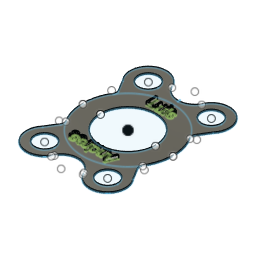
2D Plancha #1 (Autodesk Fusion 360 design; units mm, degrees)
Autodesk Fusion 360 part; units mm, degrees
sketch "Boceto1" plane through (0, 0, 0) normal (0, 0, 1) x (1, 0, 0)
  circle A0 centre (-31.4946, 51.8022) radius 10
  arc A1 (-14.8964, 58.7663) -> (-45.1155, 40.0347) centre (-31.4946, 51.8022) ccw
  line L0 (-45.1155, 40.0347) -> (-38.2984, 28.8221)
  arc A2 (-38.3137, 23.6021) -> (-38.2984, 28.8221) centre (-42.5708, 26.2246) ccw
  arc A3 (38.2984, 28.8221) -> (38.3137, 23.6021) centre (42.5708, 26.2246) ccw
  line L1 (45.1155, 40.0347) -> (38.2984, 28.8221)
  arc A4 (45.1155, 40.0347) -> (14.8964, 58.7663) centre (31.4946, 51.8022) ccw
  circle A5 centre (31.4946, 51.8022) radius 10
  arc A6 (-15.8954, 60.7834) -> (15.8954, 60.7834) centre (0, 66.8115) ccw
  line L2 (0, 49.8115) -> (0, 51.8022)
  line L3 (0, 49.8115) -> (0, 51.8022)
  arc A7 (45, 0) -> (-45, 0) centre (0, 0) ccw
  arc A8 (27.5, 0) -> (-27.5, 0) centre (0, 0) ccw
  arc A9 (-45, 0) -> (45, 0) centre (0, 0) ccw
  arc A10 (-27.5, 0) -> (27.5, 0) centre (0, 0) ccw
  line L4 (-45.1155, -40.0347) -> (-38.2984, -28.8221)
  arc A11 (-38.2984, -28.8221) -> (-38.3137, -23.6021) centre (-42.5708, -26.2246) ccw
  arc A12 (-45.1155, -40.0347) -> (-14.8964, -58.7663) centre (-31.4946, -51.8022) ccw
  circle A13 centre (-31.4946, -51.8022) radius 10
  arc A14 (15.8954, -60.7834) -> (-15.8954, -60.7834) centre (0, -66.8115) ccw
  arc A15 (14.8964, -58.7663) -> (45.1155, -40.0347) centre (31.4946, -51.8022) ccw
  circle A16 centre (31.4946, -51.8022) radius 10
  line L5 (45.1155, -40.0347) -> (38.2984, -28.8221)
  arc A17 (38.3137, -23.6021) -> (38.2984, -28.8221) centre (42.5708, -26.2246) ccw
  line L6 (-12.0362, 30.2431) -> (-12.0909, 40.2429)
  line L7 (-12.0909, 40.2429) -> (-10.7676, 40.2502)
  line L8 (-10.7676, 40.2502) -> (-10.7193, 31.4304)
  line L9 (-10.7193, 31.4304) -> (-5.7944, 31.4573)
  line L10 (-5.7944, 31.4573) -> (-5.788, 30.2773)
  line L11 (-5.788, 30.2773) -> (-12.0362, 30.2431)
  line L12 (0.3784, 30.311) -> (0.3726, 31.3751)
  spline S0 degree 2 poles (0.3726, 31.3751) (-0.4665, 30.1427) (-1.9195, 30.1347) knots 0 0 0 1 1 1
  spline S1 degree 2 poles (-1.9195, 30.1347) (-2.5606, 30.1312) (-3.1179, 30.3737) knots 0 0 0 1 1 1
  spline S2 degree 2 poles (-3.1179, 30.3737) (-3.6752, 30.6162) (-3.9467, 30.9865) knots 0 0 0 1 1 1
  spline S3 degree 2 poles (-3.9467, 30.9865) (-4.2181, 31.3568) (-4.3302, 31.8951) knots 0 0 0 1 1 1
  spline S4 degree 2 poles (-4.3302, 31.8951) (-4.4072, 32.2562) (-4.4115, 33.0406) knots 0 0 0 1 1 1
  line L13 (-4.4115, 33.0406) -> (-4.4361, 37.529)
  line L14 (-4.4361, 37.529) -> (-3.2083, 37.5357)
  line L15 (-3.2083, 37.5357) -> (-3.1863, 33.518)
  spline S5 degree 2 poles (-3.1863, 33.518) (-3.181, 32.5562) (-3.1042, 32.2224) knots 0 0 0 1 1 1
  spline S6 degree 2 poles (-3.1042, 32.2224) (-2.9855, 31.7387) (-2.6089, 31.4645) knots 0 0 0 1 1 1
  spline S7 degree 2 poles (-2.6089, 31.4645) (-2.2322, 31.1903) (-1.6797, 31.1933) knots 0 0 0 1 1 1
  spline S8 degree 2 poles (-1.6797, 31.1933) (-1.1272, 31.1964) (-0.6444, 31.4821) knots 0 0 0 1 1 1
  spline S9 degree 2 poles (-0.6444, 31.4821) (-0.1617, 31.7678) (0.0369, 32.2566) knots 0 0 0 1 1 1
  spline S10 degree 2 poles (0.0369, 32.2566) (0.2355, 32.7454) (0.2304, 33.6731) knots 0 0 0 1 1 1
  line L16 (0.2304, 33.6731) -> (0.2092, 37.5544)
  line L17 (0.2092, 37.5544) -> (1.437, 37.5611)
  line L18 (1.437, 37.5611) -> (1.4766, 30.317)
  line L19 (1.4766, 30.317) -> (0.3784, 30.311)
  line L20 (3.36, 38.9154) -> (3.3523, 40.3274)
  line L21 (3.3523, 40.3274) -> (4.5801, 40.3341)
  line L22 (4.5801, 40.3341) -> (4.5878, 38.9221)
  line L23 (4.5878, 38.9221) -> (3.36, 38.9154)
  line L24 (3.407, 30.3276) -> (3.3674, 37.5717)
  line L25 (3.3674, 37.5717) -> (4.5952, 37.5784)
  line L26 (4.5952, 37.5784) -> (4.6348, 30.3343)
  line L27 (4.6348, 30.3343) -> (3.407, 30.3276)
  line L28 (6.0009, 32.5041) -> (7.214, 32.7018)
  spline S11 degree 2 poles (7.214, 32.7018) (7.3203, 31.9725) (7.7897, 31.5862) knots 0 0 0 1 1 1
  spline S12 degree 2 poles (7.7897, 31.5862) (8.259, 31.2) (9.098, 31.2045) knots 0 0 0 1 1 1
  spline S13 degree 2 poles (9.098, 31.2045) (9.9439, 31.2092) (10.3513, 31.5559) knots 0 0 0 1 1 1
  spline S14 degree 2 poles (10.3513, 31.5559) (10.7586, 31.9026) (10.7561, 32.3664) knots 0 0 0 1 1 1
  spline S15 degree 2 poles (10.7561, 32.3664) (10.7538, 32.7825) (10.391, 33.0193) knots 0 0 0 1 1 1
  spline S16 degree 2 poles (10.391, 33.0193) (10.1377, 33.1816) (9.1336, 33.4285) knots 0 0 0 1 1 1
  spline S17 degree 2 poles (9.1336, 33.4285) (7.7812, 33.7622) (7.258, 34.0083) knots 0 0 0 1 1 1
  spline S18 degree 2 poles (7.258, 34.0083) (6.7348, 34.2544) (6.463, 34.6929) knots 0 0 0 1 1 1
  spline S19 degree 2 poles (6.463, 34.6929) (6.1911, 35.1314) (6.1882, 35.6635) knots 0 0 0 1 1 1
  spline S20 degree 2 poles (6.1882, 35.6635) (6.1856, 36.1478) (6.405, 36.5617) knots 0 0 0 1 1 1
  spline S21 degree 2 poles (6.405, 36.5617) (6.6244, 36.9756) (7.0049, 37.2505) knots 0 0 0 1 1 1
  spline S22 degree 2 poles (7.0049, 37.2505) (7.2902, 37.4635) (7.784, 37.6129) knots 0 0 0 1 1 1
  spline S23 degree 2 poles (7.784, 37.6129) (8.2777, 37.7622) (8.8439, 37.7653) knots 0 0 0 1 1 1
  spline S24 degree 2 poles (8.8439, 37.7653) (9.6965, 37.77) (10.3425, 37.528) knots 0 0 0 1 1 1
  spline S25 degree 2 poles (10.3425, 37.528) (10.9884, 37.2859) (11.2977, 36.8681) knots 0 0 0 1 1 1
  spline S26 degree 2 poles (11.2977, 36.8681) (11.6069, 36.4503) (11.7267, 35.7483) knots 0 0 0 1 1 1
  line L29 (11.7267, 35.7483) -> (10.5271, 35.5781)
  spline S27 degree 2 poles (10.5271, 35.5781) (10.4422, 36.1369) (10.0482, 36.4486) knots 0 0 0 1 1 1
  spline S28 degree 2 poles (10.0482, 36.4486) (9.6543, 36.7602) (8.9381, 36.7563) knots 0 0 0 1 1 1
  spline S29 degree 2 poles (8.9381, 36.7563) (8.0922, 36.7517) (7.7322, 36.47) knots 0 0 0 1 1 1
  spline S30 degree 2 poles (7.7322, 36.47) (7.3723, 36.1884) (7.3743, 35.8132) knots 0 0 0 1 1 1
  spline S31 degree 2 poles (7.3743, 35.8132) (7.3756, 35.5745) (7.5267, 35.3843) knots 0 0 0 1 1 1
  spline S32 degree 2 poles (7.5267, 35.3843) (7.6779, 35.1873) (7.9992, 35.0594) knots 0 0 0 1 1 1
  spline S33 degree 2 poles (7.9992, 35.0594) (8.1837, 34.9922) (9.0855, 34.7516) knots 0 0 0 1 1 1
  spline S34 degree 2 poles (9.0855, 34.7516) (10.3902, 34.4108) (10.9064, 34.192) knots 0 0 0 1 1 1
  spline S35 degree 2 poles (10.9064, 34.192) (11.4226, 33.9731) (11.7183, 33.5518) knots 0 0 0 1 1 1
  spline S36 degree 2 poles (11.7183, 33.5518) (12.0139, 33.1305) (12.0173, 32.5029) knots 0 0 0 1 1 1
  spline S37 degree 2 poles (12.0173, 32.5029) (12.0207, 31.889) (11.6655, 31.3448) knots 0 0 0 1 1 1
  spline S38 degree 2 poles (11.6655, 31.3448) (11.3104, 30.8005) (10.6367, 30.5001) knots 0 0 0 1 1 1
  spline S39 degree 2 poles (10.6367, 30.5001) (9.963, 30.1997) (9.1104, 30.1951) knots 0 0 0 1 1 1
  spline S40 degree 2 poles (9.1104, 30.1951) (7.6984, 30.1873) (6.9551, 30.7699) knots 0 0 0 1 1 1
  spline S41 degree 2 poles (6.9551, 30.7699) (6.2118, 31.3525) (6.0009, 32.5041) knots 0 0 0 1 1 1
  line L30 (20.5732, -29.8279) -> (16.7328, -39.8279)
  line L31 (16.7328, -39.8279) -> (15.3071, -39.8279)
  line L32 (15.3071, -39.8279) -> (11.2144, -29.8279)
  line L33 (11.2144, -29.8279) -> (12.7219, -29.8279)
  line L34 (12.7219, -29.8279) -> (13.8883, -32.8566)
  line L35 (13.8883, -32.8566) -> (18.0697, -32.8566)
  line L36 (18.0697, -32.8566) -> (19.168, -29.8279)
  line L37 (19.168, -29.8279) -> (20.5732, -29.8279)
  line L38 (17.6878, -33.9343) -> (14.2976, -33.9343)
  line L39 (14.2976, -33.9343) -> (15.3412, -36.7038)
  spline S42 degree 2 poles (15.3412, -36.7038) (15.8187, -37.9657) (16.0506, -38.7774) knots 0 0 0 1 1 1
  spline S43 degree 2 poles (16.0506, -38.7774) (16.2416, -37.8156) (16.5895, -36.8675) knots 0 0 0 1 1 1
  line L40 (16.5895, -36.8675) -> (17.6878, -33.9343)
  line L41 (10.3139, -29.8279) -> (10.3139, -37.0721)
  line L42 (10.3139, -37.0721) -> (9.2089, -37.0721)
  line L43 (9.2089, -37.0721) -> (9.2089, -36.0421)
  spline S44 degree 2 poles (9.2089, -36.0421) (8.4108, -37.2358) (6.9033, -37.2358) knots 0 0 0 1 1 1
  spline S45 degree 2 poles (6.9033, -37.2358) (6.2485, -37.2358) (5.6994, -37.0005) knots 0 0 0 1 1 1
  spline S46 degree 2 poles (5.6994, -37.0005) (5.1502, -36.7651) (4.8774, -36.3832) knots 0 0 0 1 1 1
  spline S47 degree 2 poles (4.8774, -36.3832) (4.6045, -36.0012) (4.4954, -35.4759) knots 0 0 0 1 1 1
  spline S48 degree 2 poles (4.4954, -35.4759) (4.4272, -35.1349) (4.4272, -34.2822) knots 0 0 0 1 1 1
  line L44 (4.4272, -34.2822) -> (4.4272, -29.8279)
  line L45 (4.4272, -29.8279) -> (5.655, -29.8279)
  line L46 (5.655, -29.8279) -> (5.655, -34.2345)
  spline S49 degree 2 poles (5.655, -34.2345) (5.655, -34.9848) (5.7983, -35.3566) knots 0 0 0 1 1 1
  spline S50 degree 2 poles (5.7983, -35.3566) (5.9415, -35.7283) (6.3064, -35.95) knots 0 0 0 1 1 1
  spline S51 degree 2 poles (6.3064, -35.95) (6.6714, -36.1717) (7.1625, -36.1717) knots 0 0 0 1 1 1
  spline S52 degree 2 poles (7.1625, -36.1717) (7.947, -36.1717) (8.5165, -35.6737) knots 0 0 0 1 1 1
  spline S53 degree 2 poles (8.5165, -35.6737) (9.0861, -35.1758) (9.0861, -33.7842) knots 0 0 0 1 1 1
  line L47 (9.0861, -33.7842) -> (9.0861, -29.8279)
  line L48 (9.0861, -29.8279) -> (10.3139, -29.8279)
  line L49 (-2.1554, -29.8279) -> (-2.1554, -30.742)
  spline S54 degree 2 poles (-2.1554, -30.742) (-1.4664, -29.6642) (-0.1294, -29.6642) knots 0 0 0 1 1 1
  spline S55 degree 2 poles (-0.1294, -29.6642) (0.7369, -29.6642) (1.4633, -30.1417) knots 0 0 0 1 1 1
  spline S56 degree 2 poles (1.4633, -30.1417) (2.1898, -30.6192) (2.5888, -31.4752) knots 0 0 0 1 1 1
  spline S57 degree 2 poles (2.5888, -31.4752) (2.9879, -32.3313) (2.9879, -33.4432) knots 0 0 0 1 1 1
  spline S58 degree 2 poles (2.9879, -33.4432) (2.9879, -34.5278) (2.6264, -35.4111) knots 0 0 0 1 1 1
  spline S59 degree 2 poles (2.6264, -35.4111) (2.2648, -36.2945) (1.5418, -36.7651) knots 0 0 0 1 1 1
  spline S60 degree 2 poles (1.5418, -36.7651) (0.8187, -37.2358) (-0.0749, -37.2358) knots 0 0 0 1 1 1
  spline S61 degree 2 poles (-0.0749, -37.2358) (-0.7297, -37.2358) (-1.2413, -36.9596) knots 0 0 0 1 1 1
  spline S62 degree 2 poles (-1.2413, -36.9596) (-1.7529, -36.6833) (-2.0735, -36.2399) knots 0 0 0 1 1 1
  line L50 (-2.0735, -36.2399) -> (-2.0735, -39.8279)
  line L51 (-2.0735, -39.8279) -> (-3.2945, -39.8279)
  line L52 (-3.2945, -39.8279) -> (-3.2945, -29.8279)
  line L53 (-3.2945, -29.8279) -> (-2.1554, -29.8279)
  spline S63 degree 2 poles (1.726, -33.4432) (1.726, -32.0516) (1.1393, -31.3627) knots 0 0 0 1 1 1
  spline S64 degree 2 poles (1.1393, -31.3627) (0.5527, -30.6737) (-0.2454, -30.6737) knots 0 0 0 1 1 1
  spline S65 degree 2 poles (-0.2454, -30.6737) (-1.0503, -30.6737) (-1.6131, -31.332) knots 0 0 0 1 1 1
  spline S66 degree 2 poles (-1.6131, -31.332) (-2.1758, -31.9902) (-2.1758, -33.3409) knots 0 0 0 1 1 1
  spline S67 degree 2 poles (-2.1758, -33.3409) (-2.1758, -34.8279) (-1.6028, -35.5237) knots 0 0 0 1 1 1
  spline S68 degree 2 poles (-1.6028, -35.5237) (-1.0298, -36.2194) (-0.1908, -36.2194) knots 0 0 0 1 1 1
  spline S69 degree 2 poles (-0.1908, -36.2194) (0.6277, -36.2194) (1.1768, -35.551) knots 0 0 0 1 1 1
  spline S70 degree 2 poles (1.1768, -35.551) (1.726, -34.8825) (1.726, -33.4432) knots 0 0 0 1 1 1
  line L54 (-5.2113, -29.8279) -> (-5.2113, -37.0721)
  line L55 (-5.2113, -37.0721) -> (-6.3163, -37.0721)
  line L56 (-6.3163, -37.0721) -> (-6.3163, -35.9739)
  spline S71 degree 2 poles (-6.3163, -35.9739) (-6.7393, -36.7447) (-7.0974, -36.9902) knots 0 0 0 1 1 1
  spline S72 degree 2 poles (-7.0974, -36.9902) (-7.4555, -37.2358) (-7.8852, -37.2358) knots 0 0 0 1 1 1
  spline S73 degree 2 poles (-7.8852, -37.2358) (-8.506, -37.2358) (-9.1472, -36.8402) knots 0 0 0 1 1 1
  line L57 (-9.1472, -36.8402) -> (-8.7243, -35.701)
  spline S74 degree 2 poles (-8.7243, -35.701) (-8.274, -35.9671) (-7.8238, -35.9671) knots 0 0 0 1 1 1
  spline S75 degree 2 poles (-7.8238, -35.9671) (-7.4214, -35.9671) (-7.1008, -35.7249) knots 0 0 0 1 1 1
  spline S76 degree 2 poles (-7.1008, -35.7249) (-6.7802, -35.4827) (-6.6438, -35.053) knots 0 0 0 1 1 1
  spline S77 degree 2 poles (-6.6438, -35.053) (-6.4391, -34.3982) (-6.4391, -33.6205) knots 0 0 0 1 1 1
  line L58 (-6.4391, -33.6205) -> (-6.4391, -29.8279)
  line L59 (-6.4391, -29.8279) -> (-5.2113, -29.8279)
  line L60 (-14.8361, -32.1608) -> (-16.1049, -32.0039)
  spline S78 degree 2 poles (-16.1049, -32.0039) (-15.8047, -30.892) (-14.993, -30.2781) knots 0 0 0 1 1 1
  spline S79 degree 2 poles (-14.993, -30.2781) (-14.1813, -29.6642) (-12.9193, -29.6642) knots 0 0 0 1 1 1
  spline S80 degree 2 poles (-12.9193, -29.6642) (-11.33, -29.6642) (-10.3989, -30.643) knots 0 0 0 1 1 1
  spline S81 degree 2 poles (-10.3989, -30.643) (-9.4678, -31.6219) (-9.4678, -33.3886) knots 0 0 0 1 1 1
  spline S82 degree 2 poles (-9.4678, -33.3886) (-9.4678, -35.2167) (-10.4091, -36.2263) knots 0 0 0 1 1 1
  spline S83 degree 2 poles (-10.4091, -36.2263) (-11.3504, -37.2358) (-12.8511, -37.2358) knots 0 0 0 1 1 1
  spline S84 degree 2 poles (-12.8511, -37.2358) (-14.3041, -37.2358) (-15.2249, -36.2467) knots 0 0 0 1 1 1
  spline S85 degree 2 poles (-15.2249, -36.2467) (-16.1458, -35.2576) (-16.1458, -33.4636) knots 0 0 0 1 1 1
  spline S86 degree 2 poles (-16.1458, -33.4636) (-16.1458, -33.3545) (-16.139, -33.1362) knots 0 0 0 1 1 1
  line L61 (-16.139, -33.1362) -> (-10.7365, -33.1362)
  spline S87 degree 2 poles (-10.7365, -33.1362) (-10.8047, -31.9425) (-11.4118, -31.3081) knots 0 0 0 1 1 1
  spline S88 degree 2 poles (-11.4118, -31.3081) (-12.0189, -30.6737) (-12.9262, -30.6737) knots 0 0 0 1 1 1
  spline S89 degree 2 poles (-12.9262, -30.6737) (-13.6015, -30.6737) (-14.079, -31.0284) knots 0 0 0 1 1 1
  spline S90 degree 2 poles (-14.079, -31.0284) (-14.5564, -31.3832) (-14.8361, -32.1608) knots 0 0 0 1 1 1
  line L62 (-10.8047, -34.1458) -> (-14.8498, -34.1458)
  spline S91 degree 2 poles (-14.8498, -34.1458) (-14.7679, -35.0598) (-14.3859, -35.5169) knots 0 0 0 1 1 1
  spline S92 degree 2 poles (-14.3859, -35.5169) (-13.7993, -36.2263) (-12.8648, -36.2263) knots 0 0 0 1 1 1
  spline S93 degree 2 poles (-12.8648, -36.2263) (-12.0189, -36.2263) (-11.4425, -35.6601) knots 0 0 0 1 1 1
  spline S94 degree 2 poles (-11.4425, -35.6601) (-10.8661, -35.0939) (-10.8047, -34.1458) knots 0 0 0 1 1 1
  line L63 (-17.1554, -31.9902) -> (-18.3695, -32.1812)
  spline S95 degree 2 poles (-18.3695, -32.1812) (-18.4719, -31.4514) (-18.9391, -31.0626) knots 0 0 0 1 1 1
  spline S96 degree 2 poles (-18.9391, -31.0626) (-19.4064, -30.6737) (-20.2454, -30.6737) knots 0 0 0 1 1 1
  spline S97 degree 2 poles (-20.2454, -30.6737) (-21.0912, -30.6737) (-21.5005, -31.0182) knots 0 0 0 1 1 1
  spline S98 degree 2 poles (-21.5005, -31.0182) (-21.9098, -31.3627) (-21.9098, -31.8265) knots 0 0 0 1 1 1
  spline S99 degree 2 poles (-21.9098, -31.8265) (-21.9098, -32.2426) (-21.5483, -32.4814) knots 0 0 0 1 1 1
  spline S100 degree 2 poles (-21.5483, -32.4814) (-21.2959, -32.6451) (-20.2931, -32.8975) knots 0 0 0 1 1 1
  spline S101 degree 2 poles (-20.2931, -32.8975) (-18.9425, -33.2385) (-18.4207, -33.4875) knots 0 0 0 1 1 1
  spline S102 degree 2 poles (-18.4207, -33.4875) (-17.8989, -33.7365) (-17.6294, -34.1765) knots 0 0 0 1 1 1
  spline S103 degree 2 poles (-17.6294, -34.1765) (-17.36, -34.6164) (-17.36, -35.1485) knots 0 0 0 1 1 1
  spline S104 degree 2 poles (-17.36, -35.1485) (-17.36, -35.6328) (-17.5817, -36.0455) knots 0 0 0 1 1 1
  spline S105 degree 2 poles (-17.5817, -36.0455) (-17.8034, -36.4582) (-18.1854, -36.731) knots 0 0 0 1 1 1
  spline S106 degree 2 poles (-18.1854, -36.731) (-18.4719, -36.9425) (-18.9664, -37.0892) knots 0 0 0 1 1 1
  spline S107 degree 2 poles (-18.9664, -37.0892) (-19.4609, -37.2358) (-20.0271, -37.2358) knots 0 0 0 1 1 1
  spline S108 degree 2 poles (-20.0271, -37.2358) (-20.8798, -37.2358) (-21.5244, -36.9902) knots 0 0 0 1 1 1
  spline S109 degree 2 poles (-21.5244, -36.9902) (-22.169, -36.7447) (-22.476, -36.3252) knots 0 0 0 1 1 1
  spline S110 degree 2 poles (-22.476, -36.3252) (-22.7829, -35.9057) (-22.8989, -35.2031) knots 0 0 0 1 1 1
  line L64 (-22.8989, -35.2031) -> (-21.6983, -35.0394)
  spline S111 degree 2 poles (-21.6983, -35.0394) (-21.6165, -35.5987) (-21.2243, -35.9125) knots 0 0 0 1 1 1
  spline S112 degree 2 poles (-21.2243, -35.9125) (-20.832, -36.2263) (-20.1158, -36.2263) knots 0 0 0 1 1 1
  spline S113 degree 2 poles (-20.1158, -36.2263) (-19.27, -36.2263) (-18.9084, -35.9466) knots 0 0 0 1 1 1
  spline S114 degree 2 poles (-18.9084, -35.9466) (-18.5469, -35.6669) (-18.5469, -35.2918) knots 0 0 0 1 1 1
  spline S115 degree 2 poles (-18.5469, -35.2918) (-18.5469, -35.053) (-18.697, -34.862) knots 0 0 0 1 1 1
  spline S116 degree 2 poles (-18.697, -34.862) (-18.847, -34.6642) (-19.1676, -34.5346) knots 0 0 0 1 1 1
  spline S117 degree 2 poles (-19.1676, -34.5346) (-19.3518, -34.4664) (-20.2522, -34.2208) knots 0 0 0 1 1 1
  spline S118 degree 2 poles (-20.2522, -34.2208) (-21.5551, -33.8729) (-22.0701, -33.6512) knots 0 0 0 1 1 1
  spline S119 degree 2 poles (-22.0701, -33.6512) (-22.5851, -33.4295) (-22.8784, -33.0066) knots 0 0 0 1 1 1
  spline S120 degree 2 poles (-22.8784, -33.0066) (-23.1717, -32.5837) (-23.1717, -31.9561) knots 0 0 0 1 1 1
  spline S121 degree 2 poles (-23.1717, -31.9561) (-23.1717, -31.3422) (-22.8136, -30.7999) knots 0 0 0 1 1 1
  spline S122 degree 2 poles (-22.8136, -30.7999) (-22.4555, -30.2576) (-21.7802, -29.9609) knots 0 0 0 1 1 1
  spline S123 degree 2 poles (-21.7802, -29.9609) (-21.1049, -29.6642) (-20.2522, -29.6642) knots 0 0 0 1 1 1
  spline S124 degree 2 poles (-20.2522, -29.6642) (-18.8402, -29.6642) (-18.1001, -30.2508) knots 0 0 0 1 1 1
  spline S125 degree 2 poles (-18.1001, -30.2508) (-17.36, -30.8375) (-17.1554, -31.9902) knots 0 0 0 1 1 1
  constraint coincident A7.centre A8.centre
  constraint concentric A7 A8
  constraint concentric A0 A1
  constraint tangent L0 A2
  constraint tangent A2 A7
  constraint coincident A2.start A7
  constraint coincident A1 A6.start
  constraint coincident A4 A6.end
  constraint coincident A6 L2.start
extrude "Extruir1" add sketch "Boceto1" along normal blind 0.01 contours A1 L0 A2 A3 L1 A4 A6 A7 | A7 A9 | A9 L4 A11 A12 A14 A15 L5 A17 | L6 L7 L8 L9 L10 L11 | L12 S0 S1 S2 S3 S4 L13 L14 L15 S5 S6 S7 S8 S9 S10 L16 L17 L18 L19 | L20 L21 L22 L23 | L24 L25 L26 L27 | L28 S11 S12 S13 S14 S15 S16 S17 S18 S19 S20 S21 S22 S23 S24 S25 S26 L29 S27 S28 S29 S30 S31 S32 S33 S34 S35 S36 S37 S38 S39 S40 S41 | L30 L31 L32 L33 L34 L35 L36 L37 | L38 L39 S42 S43 L40 | L41 L42 L43 S44 S45 S46 S47 S48 L44 L45 L46 S49 S50 S51 S52 S53 L47 L48 | L49 S54 S55 S56 S57 S58 S59 S60 S61 S62 L50 L51 L52 L53 | S63 S64 S65 S66 S67 S68 S69 S70 | L54 L55 L56 S71 S72 S73 L57 S74 S75 S76 S77 L58 L59 | L60 S78 S79 S80 S81 S82 S83 S84 S85 S86 L61 S87 S88 S89 S90 | L62 S91 S92 S93 S94 | L63 S95 S96 S97 S98 S99 S100 S101 S102 S103 S104 S105 S106 S107 S108 S109 S110 L64 S111 S112 S113 S114 S115 S116 S117 S118 S119 S120 S121 S122 S123 S124 S125 makes body 1
extrude "Extruir2" add 1 faces at (11.7556, -41.2844, 0.01) along direction (0, 0, 1) blind 1 on bodies 1 bodies 1
extrude "Extruir3" add sketch "Boceto1" along normal blind 4 separate body contours L6 L7 L8 L9 L10 L11 | L12 S0 S1 S2 S3 S4 L13 L14 L15 S5 S6 S7 S8 S9 S10 L16 L17 L18 L19 | L20 L21 L22 L23 | L24 L25 L26 L27 | L28 S11 S12 S13 S14 S15 S16 S17 S18 S19 S20 S21 S22 S23 S24 S25 S26 L29 S27 S28 S29 S30 S31 S32 S33 S34 S35 S36 S37 S38 S39 S40 S41 | L30 L31 L32 L33 L34 L35 L36 L37 | L41 L42 L43 S44 S45 S46 S47 S48 L44 L45 L46 S49 S50 S51 S52 S53 L47 L48 | L49 S54 S55 S56 S57 S58 S59 S60 S61 S62 L50 L51 L52 L53 | L54 L55 L56 S71 S72 S73 L57 S74 S75 S76 S77 L58 L59 | L60 S78 S79 S80 S81 S82 S83 S84 S85 S86 L61 S87 S88 S89 S90 | L63 S95 S96 S97 S98 S99 S100 S101 S102 S103 S104 S105 S106 S107 S108 S109 S110 L64 S111 S112 S113 S114 S115 S116 S117 S118 S119 S120 S121 S122 S123 S124 S125 makes body 2 at (4.6084, 35.1637, 1.3333) makes body 3 at (10.3139, -32.2426, 1.3333) makes body 4 at (-21.0999, -33.527, 0) makes body 5 at (-3.2945, -36.4946, 1.3333) makes body 6 at (1.4502, 35.1464, 1.3333) makes body 7 at (3.3574, 39.3861, 1.3333) makes body 8 at (-12.0544, 33.5764, 1.3333) makes body 9 at (-13.9084, -33.4727, 0) makes body 10 at (-5.2113, -32.2426, 1.3333) makes body 11 at (13.9429, -36.4946, 1.3333) makes body 12 at (9.937, 34.0625, 0)
extrude "Extruir4" add sketch "Boceto1" along normal blind 1 contours A1 L0 A2 A3 L1 A4 A6 A7 | A7 A9 | A9 L4 A11 A12 A14 A15 L5 A17 bodies 2 3 4 5 6 7 8 9 10 11 12
hidden bodies 1
